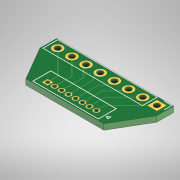
# Autodesk Inventor part: board_display
Saved by Autodesk Inventor 2022.2 (Build 262287010, 287A)
## iProperties
Created: 2026-01-01
Part Number: board_display
Material: Generic
Document SubType Name: Modeling
Designer: dbstj
Density: 1 g/cm^3
Appearance: Default
Author: dbstj
Autodesk Inventor part; units mm, degrees
ref_plane "YZ Plane" through (0, 0, 0) normal (1, 0, 0) x (0, 1, 0)
ref_plane "XZ Plane" through (0, 0, 0) normal (0, 1, 0) x (-1, 0, 0)
ref_plane "XY Plane" through (0, 0, 0) normal (0, 0, 1) x (1, 0, 0)
sketch "스케치1" plane through (0, 0, 0) normal (0, 1, 0) x (-1, 0, 0)
  line L0 (10.5, 4.5) -> (-10.5, 4.5)
  line L1 (-10.5, 4.5) -> (-10.5, -4.5)
  line L2 (-10.5, -4.5) -> (10.5, -4.5)
  line L3 (10.5, -4.5) -> (10.5, 4.5)
  line L4 (10.5, 4.5) -> (-10.5, -4.5) construction
  line L5 (-10.5, 4.5) -> (10.5, -4.5) construction
  point P0 (0, 0)
  dimension "d0" = 21
  dimension "d1" = 9
  constraints: 12 end point, 2 midpoint, 2 parallel, 1 horizontal, 1 perpendicular
  measures "d0" distance of L2.end L1.end
  measures "d1" distance of L1.end L0.end
extrude "돌출1" add sketch "스케치1" along normal blind 1
sketch "스케치2" plane through (0, 1, 0) normal (0, 1, 0) x (1, 0, 0)
  line L0 (10.5, 4.5) -> (-10.5, 4.5) projected
  line L1 (10.5, -4.5) -> (10.5, 4.5) projected
  line L2 (-10.5, -4.5) -> (10.5, -4.5) projected
  point P0 (0, 0)
  point P1 (1.28, 3.1)
  point P2 (3.82, 3.1)
  point P3 (6.36, 3.1)
  point P4 (8.9, 3.1)
  point P5 (-1.26, 3.1)
  point P6 (-3.8, 3.1)
  point P7 (-6.34, 3.1)
  point P8 (-8.88, 3.1)
  point P9 (0.5, -3.1)
  point P10 (1.75, -3.1)
  point P11 (3, -3.1)
  point P12 (4.25, -3.1)
  point P13 (-0.75, -3.1)
  point P14 (-2, -3.1)
  point P15 (-3.25, -3.1)
  point P16 (-4.5, -3.1)
  dimension "d4" = 2.54
  dimension "d5" = 2.54
  dimension "d6" = 2.54
  dimension "d7" = 2.54
  dimension "d8" = 2.54
  dimension "d9" = 2.54
  dimension "d10" = 2.54
  dimension "d11" = 1.4
  dimension "d13" = 1.25
  dimension "d15" = 1.25
  dimension "d16" = 1.25
  dimension "d17" = 1.25
  dimension "d18" = 1.25
  dimension "d19" = 1.25
  dimension "d20" = 1.25
  dimension "d23" = 6.2
  dimension "d45" = 1.6
  dimension "d142" = 15
  constraints: 14 horizontal alignment
  measures "d4" distance of point (6.36, 3.1) point (8.9, 3.1)
  measures "d5" distance of point (3.82, 3.1) point (6.36, 3.1)
  measures "d6" distance of point (1.28, 3.1) point (3.82, 3.1)
  measures "d7" distance of point (-1.26, 3.1) point (1.28, 3.1)
  measures "d8" distance of point (-3.8, 3.1) point (-1.26, 3.1)
  measures "d9" distance of point (-6.34, 3.1) point (-3.8, 3.1)
  measures "d10" distance of point (-8.88, 3.1) point (-6.34, 3.1)
  measures "d11" distance from line of L0 point (8.9, 3.1)
  measures "d13" distance of point (3, -3.1) point (4.25, -3.1)
  measures "d15" distance of point (3, -3.1) point (1.75, -3.1)
  measures "d16" distance of point (0.5, -3.1) point (1.75, -3.1)
  measures "d17" distance of point (-0.75, -3.1) point (0.5, -3.1)
  measures "d18" distance of point (-2, -3.1) point (-0.75, -3.1)
  measures "d19" distance of point (-2, -3.1) point (-3.25, -3.1)
  measures "d20" distance of point (-4.5, -3.1) point (-3.25, -3.1)
  measures "d23" vertical distance of point (4.25, -3.1) point (8.9, 3.1)
  measures "d45" distance from line of L1 point (8.9, 3.1)
  measures "d142" distance from line of L1 point (-4.5, -3.1)
hole "구멍1" at (-8.88, 1, -3.1) at (-6.34, 1, -3.1) at (-3.8, 1, -3.1) at (-1.26, 1, -3.1) at (8.9, 1, -3.1) at (6.36, 1, -3.1) at (3.82, 1, -3.1) at (1.28, 1, -3.1) direction (0, -1, 0) diameter 1 end through all
hole "구멍2" at (0.5, 1, 3.1) at (1.75, 1, 3.1) at (3, 1, 3.1) at (4.25, 1, 3.1) at (-0.75, 1, 3.1) at (-2, 1, 3.1) at (-3.25, 1, 3.1) at (-4.5, 1, 3.1) direction (0, -1, 0) diameter 0.6 end through all
sketch "스케치3" plane through (0, 1, 0) normal (0, 1, 0) x (1, 0, 0)
  line L0 (-10.5, -4.5) -> (10.5, -4.5) projected
  line L1 (7, -4.5) -> (10.5, 1.5)
  line L2 (10.5, -4.5) -> (10.5, 4.5) projected
  line L3 (-7, -4.5) -> (-10.5, 1.5)
  line L4 (-10.5, 4.5) -> (-10.5, -4.5) projected
  point P0 (0, 0)
  dimension "d38" = 7
  dimension "d39" = 7
  dimension "d40" = 3
  dimension "d41" = 3
  dimension "d44" = 3.5
  constraints: 4 end point, 4 point on line
  measures "d38" horizontal distance of point (0, 0) L1.start
  measures "d39" horizontal distance of point (0, 0) L3.start
  measures "d40" distance of L4.start L3.end
  measures "d41" distance of L2.end L1.end
  measures "d44" distance of L0.end L1.start
extrude "돌출2" cut sketch "스케치3" against normal blind 1
sketch "스케치4" plane through (0, 1, 0) normal (0, 1, 0) x (1, 0, 0)
  line L0 (7, -4.5) -> (10.5, 1.5) projected
  line L1 (10.5, 1.5) -> (10.5, 4.5) projected
  line L2 (10.5, 4.5) -> (-10.5, 4.5) projected
  line L3 (-10.5, 4.5) -> (-10.5, 1.5) projected
  line L4 (-10.5, 1.5) -> (-7, -4.5) projected
  line L5 (-7, -4.5) -> (7, -4.5) projected
  circle A0 centre (-3.25, -3.1) radius 0.3 projected
  circle A1 centre (-0.75, -3.1) radius 0.3 projected
  circle A2 centre (3, -3.1) radius 0.3 projected
  circle A3 centre (0.5, -3.1) radius 0.3 projected
  circle A4 centre (1.75, -3.1) radius 0.3 projected
  circle A5 centre (4.25, -3.1) radius 0.3 projected
  circle A6 centre (-2, -3.1) radius 0.3 projected
  circle A7 centre (-4.5, -3.1) radius 0.3 projected
  circle A8 centre (3.82, 3.1) radius 0.5 projected
  circle A9 centre (8.9, 3.1) radius 0.5 projected
  circle A10 centre (-3.8, 3.1) radius 0.5 projected
  circle A11 centre (-8.88, 3.1) radius 0.5 projected
  circle A12 centre (-6.34, 3.1) radius 0.5 projected
  circle A13 centre (-1.26, 3.1) radius 0.5 projected
  circle A14 centre (6.36, 3.1) radius 0.5 projected
  circle A15 centre (1.28, 3.1) radius 0.5 projected
  line L6 (-7, -4.5) -> (7, -4.5) projected
  line L7 (-10.5712, 4.607) -> (10.5945, 4.607) construction
  line L8 (10.5945, 4.607) -> (10.5945, -4.5865) construction
  line L9 (10.5945, -4.5865) -> (-10.5712, -4.5865) construction
  line L10 (-10.5712, -4.5865) -> (-10.5712, 4.607) construction
  line L11 (10.5, 4.5) -> (-10.5, 4.5) projected
  point P0 (0, 0)
  constraints: 1 parallel, 2 other
decal "전사1"
sketch "스케치5" plane through (0, 0, 0) normal (0, -1, 0) x (1, 0, 0)
  line L0 (10.5, -1.5) -> (7, 4.5) projected
  line L1 (-7, 4.5) -> (7, 4.5) projected
  line L2 (-7, 4.5) -> (-10.5, -1.5) projected
  line L3 (-10.5, -4.5) -> (-10.5, -1.5) projected
  line L4 (10.5, -4.5) -> (-10.5, -4.5) projected
  line L5 (10.5, -1.5) -> (10.5, -4.5) projected
  circle A0 centre (-3.25, 3.1) radius 0.3 projected
  circle A1 centre (-0.75, 3.1) radius 0.3 projected
  circle A2 centre (3, 3.1) radius 0.3 projected
  circle A3 centre (0.5, 3.1) radius 0.3 projected
  circle A4 centre (1.75, 3.1) radius 0.3 projected
  circle A5 centre (4.25, 3.1) radius 0.3 projected
  circle A6 centre (-2, 3.1) radius 0.3 projected
  circle A7 centre (-4.5, 3.1) radius 0.3 projected
  circle A8 centre (3.82, -3.1) radius 0.5 projected
  circle A9 centre (8.9, -3.1) radius 0.5 projected
  circle A10 centre (-3.8, -3.1) radius 0.5 projected
  circle A11 centre (-8.88, -3.1) radius 0.5 projected
  circle A12 centre (-6.34, -3.1) radius 0.5 projected
  circle A13 centre (-1.26, -3.1) radius 0.5 projected
  circle A14 centre (6.36, -3.1) radius 0.5 projected
  circle A15 centre (1.28, -3.1) radius 0.5 projected
  line L6 (10.5, -4.5) -> (-10.5, -4.5) projected
  line L7 (10.5787, -4.5949) -> (-10.5959, -4.5949) construction
  line L8 (-10.5959, -4.5949) -> (-10.5959, 4.5842) construction
  line L9 (-10.5959, 4.5842) -> (10.5787, 4.5842) construction
  line L10 (10.5787, 4.5842) -> (10.5787, -4.5949) construction
  point P0 (0, 0)
  constraints: 1 parallel, 2 other
decal "전사2"
equation "\"d5\" = d4"
equation "\"d6\" = d4"
equation "\"d7\" = d4"
equation "\"d8\" = d4"
equation "\"d9\" = d4"
equation "\"d10\" = d4"
equation "\"d15\" = d13"
equation "\"d16\" = d13"
equation "\"d17\" = d13"
equation "\"d18\" = d13"
equation "\"d19\" = d13"
equation "\"d20\" = d13"
